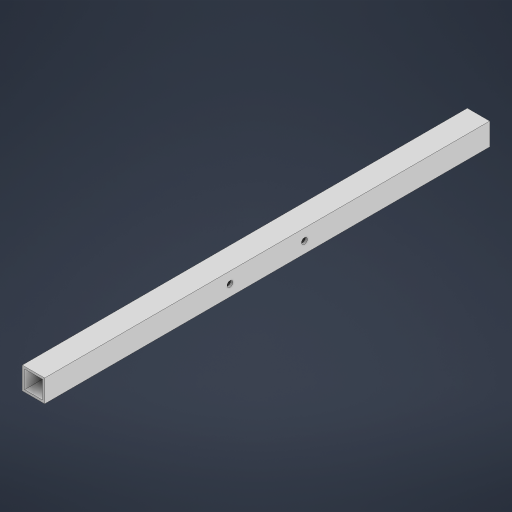
# Autodesk Inventor part: S_horizontal
Saved by Autodesk Inventor 2024 (Build 280153000, 153)
## iProperties
Created: 2023-05-17
Part Number: S_horizontal
Material: Genérico
Document SubType Name: Modeling
Designer: javie
Density: 1 g/cm^3
Appearance: Valor por defecto
Author: javie
Autodesk Inventor part; units mm, degrees
ref_plane "YZ Plane" through (0, 0, 0) normal (1, 0, 0) x (0, 1, 0)
ref_plane "XZ Plane" through (0, 0, 0) normal (0, 1, 0) x (-1, 0, 0)
ref_plane "XY Plane" through (0, 0, 0) normal (0, 0, 1) x (1, 0, 0)
sketch "Boceto1" plane through (0, 0, 0) normal (0, 0, 1) x (1, 0, 0)
  line L0 (-0.534, 0.5518) -> (14.466, 0.5518)
  line L1 (14.466, 0.5518) -> (14.466, -14.4482)
  line L2 (14.466, -14.4482) -> (-0.534, -14.4482)
  line L3 (-0.534, -14.4482) -> (-0.534, 0.5518)
  line L4 (0.966, -0.9482) -> (12.966, -0.9482)
  line L5 (12.966, -0.9482) -> (12.966, -12.9482)
  line L6 (12.966, -12.9482) -> (0.966, -12.9482)
  line L7 (0.966, -12.9482) -> (0.966, -0.9482)
  point P0 (0, 0)
  point P1 (6.966, -0.9482)
  dimension "d0" = 15
  dimension "d1" = 15
  dimension "d2" = 1.5
  dimension "d3" = 1.5
  dimension "d4" = 1.5
  dimension "d5" = 1.5
  constraints: 16 end point, 4 parallel, 2 horizontal, 2 perpendicular, 1 midpoint
  measures "d0" distance of L1.end L2.end
  measures "d1" distance of L0.end L1.end
  measures "d2" distance from line of L0 point (6.966, -0.948)
  measures "d3" distance between parallel lines of L1 L5
  measures "d4" distance between parallel lines of L3 L7
  measures "d5" distance between parallel lines of L2 L6
extrude "Extrusión1" add sketch "Boceto1" along normal blind 298.4
sketch "Boceto2" plane through (14.466, -14.4482, 0) normal (1, 0, 0) x (0, 0, -1)
  circle A0 centre (-174.2, 7.5) radius 2
  circle A1 centre (-124.2, 7.5) radius 2
  line L0 (0, 0) -> (-298.4, 0) projected
  line L1 (0, 0) -> (0, 15) projected
  point P0 (0, 14.4482)
  dimension "d8" = 4
  dimension "d9" = 4
  dimension "d10" = 7.5
  dimension "d11" = 7.5
  dimension "d12" = 50
  dimension "d13" = 124.2
  constraints: 2 centre point
  measures "d8" diameter of A0
  measures "d9" diameter of A1
  measures "d10" distance from line of L0 A0.centre
  measures "d11" distance from line of L0 A1.centre
  measures "d12" distance of A1.centre A0.centre
  measures "d13" distance from line of L1 A1.centre
extrude "Extrusión2" cut sketch "Boceto2" against normal blind 10
sketch "Boceto3" plane through (-0.534, -14.4482, 0) normal (-1, 0, 0) x (0, 0, 1)
  circle A0 centre (99.2, 7.5) radius 2
  circle A1 centre (199.2, 7.5) radius 2
  line L0 (0, 15) -> (0, 0) projected
  point P0 (0, 14.4482)
  dimension "d16" = 4
  dimension "d17" = 4
  dimension "d18" = 100
  dimension "d19" = 99.2
  constraints: 2 centre point
  measures "d16" diameter of A0
  measures "d17" diameter of A1
  measures "d18" distance of A0.centre A1.centre
  measures "d19" distance from line of L0 A0.centre
extrude "Extrusión3" cut sketch "Boceto3" against normal blind 10
